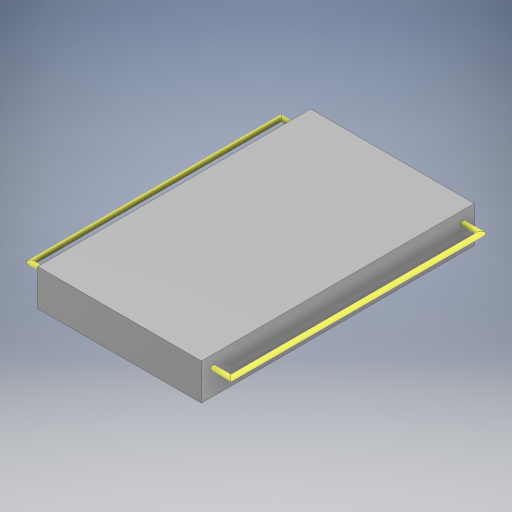
# Autodesk Inventor part: ATQ-36-60-B
Saved by Autodesk Inventor 2024.2 (Build 282272000, 272)
## iProperties
RuleStatus: InUse
Created: 2024-03-05
Part Number: ATQ-36-60-B
Material: Generic
Document SubType Name: Modeling
Designer: TiffanyHayden
Density: 1 g/cm^3
Appearance: Default
MODEL: ATQ-36-60-B
Author: TiffanyHayden
Autodesk Inventor part; units mm, degrees
ref_plane "PLANE IN" through (0, 0, 0) normal (0, 1, 0) x (-1, 0, 0)
ref_plane "PLANE OUT" through (0, 1524, 0) normal (0, 1, 0) x (-1, 0, 0)
ref_plane "PLANE CTR" through (0, 0, 0) normal (1, 0, 0) x (0, 1, 0)
ref_plane "PLANE RH" through (457.2, 0, 0) normal (1, 0, 0) x (0, 1, 0)
ref_plane "PLANE LH" through (-457.2, 0, 0) normal (1, 0, 0) x (0, 1, 0)
ref_plane "PLANE TOP" through (0, 0, 0) normal (0, 0, 1) x (1, 0, 0)
ref_plane "PLANE BOT" through (0, 0, -203.2) normal (0, 0, 1) x (1, 0, 0)
ref_plane "PLANE HANDLE RH" through (558.8, 0, 0) normal (1, 0, 0) x (0, 1, 0)
ref_plane "PLANE HANDLE LH" through (-558.8, 0, 0) normal (1, 0, 0) x (0, 1, 0)
ref_plane "PLANE HANDLE IN" through (0, 63.5, 0) normal (0, 1, 0) x (-1, 0, 0)
ref_plane "PLANE HANDLE OUT" through (0, 1460.5, 0) normal (0, 1, 0) x (-1, 0, 0)
ref_plane "PLANE HANDLE TOP" through (0, 0, -63.5) normal (0, 0, 1) x (1, 0, 0)
sketch "SKETCH BODY" plane through (0, 0, 0) normal (0, 0, 1) x (1, 0, 0)
  line L0 (-457.2, 0) -> (457.2, 0)
  line L1 (457.2, 0) -> (457.2, 1524)
  line L2 (457.2, 1524) -> (-457.2, 1524)
  line L3 (-457.2, 1524) -> (-457.2, 0)
  line L4 (-640.08, 0) -> (640.08, 0) projected
  line L5 (-640.08, 1524) -> (640.08, 1524) projected
  line L6 (457.2, 3657.6) -> (457.2, -609.6) projected
  line L7 (-457.2, 3657.6) -> (-457.2, -609.6) projected
  constraints: 8 end point, 4 collinear, 2 parallel, 1 horizontal, 1 perpendicular
extrude "EXT BODY" add sketch "SKETCH BODY" against normal blind 203.2
sketch "SKETCH HANDLE DIA" plane through (457.2, 0, 0) normal (1, 0, 0) x (0, 1, 0)
  line L0 (45.72, -63.5) -> (81.28, -63.5) projected
  line L1 (63.5, -45.72) -> (63.5, -81.28) projected
  circle A0 centre (63.5, -63.5) radius 12.7
  dimension "d79" = 25.4
  constraints: 2 midpoint, 1 centre point
  measures "d79" diameter of A0
sketch "SKETCH HANDLE PATH" plane through (0, 0, -63.5) normal (0, 0, 1) x (1, 0, 0)
  line L0 (558.8, 3568.7) -> (558.8, -520.7) projected
  line L1 (457.2, 3568.7) -> (457.2, -520.7) projected
  line L2 (436.88, 63.5) -> (579.12, 63.5) projected
  line L3 (436.88, 1460.5) -> (579.12, 1460.5) projected
  line L4 (457.2, 63.5) -> (558.8, 63.5)
  line L5 (558.8, 63.5) -> (558.8, 1460.5)
  line L6 (558.8, 1460.5) -> (457.2, 1460.5)
  line L7 (457.2, 1460.5) -> (457.2, 63.5) construction
  constraints: 8 end point, 4 collinear, 2 parallel, 1 horizontal, 1 perpendicular
sweep "SWP HANDLE" add profiles "SKETCH HANDLE DIA" path "SKETCH HANDLE PATH" path curves L4 L5 L6
mirror "MIR HANDLE" about plane through (0, 0, 0) normal (1, 0, 0)
equation "\"d76\" = HEIGHT"
equation "\"PLANE_OUT\" = LENGTH"
equation "\"PLANE_RH\" = 0.5 * WIDTH"
equation "\"PLANE_LH\" = -0.5 * WIDTH"
equation "\"PLANE_BOT\" = -HEIGHT"
equation "\"PLANE_HANDLE_RH\" = HANDLE_OFFSET_CTR"
equation "\"PLANE_HANDLE_LH\" = -HANDLE_OFFSET_CTR"
equation "\"PLANE_HANDLE_IN\" = HANDLE_OFFSET_END"
equation "\"PLANE_HANDLE_OUT\" = LENGTH - HANDLE_OFFSET_END"
equation "\"PLANE_HANDLE_TOP\" = -HANDLE_OFFSET_TOP"
equation "\"LENGTH\" = 1524"
equation "\"WIDTH\" = 914.4"
equation "\"HEIGHT\" = 203.2"
equation "\"HANDLE_GAP\" = 101.6"
equation "\"HANDLE_OFFSET_CTR\" = 0.5 * WIDTH + HANDLE_GAP"
equation "\"HANDLE_OFFSET_END\" = 63.5"
equation "\"HANDLE_OFFSET_TOP\" = 63.5"
body "Solid5"
